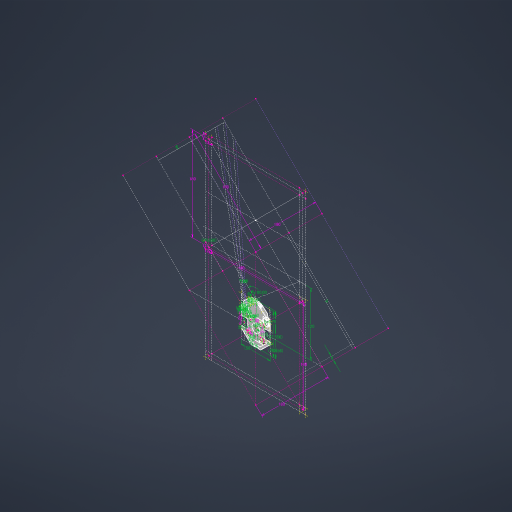
# Autodesk Inventor part: chassis
Saved by Autodesk Inventor 2023.5 (Build 275446000, 446)
## iProperties
Created: 2024-12-08
Part Number: chassis
Material: 一般
Document SubType Name: Modeling
Designer: IshiiLabHonda
Density: 1 g/cm^3
Appearance: 既定
Author: IshiiLabHonda
Autodesk Inventor part; units mm, degrees
(part 1 of 2)
ref_plane "YZ Plane" through (0, 0, 0) normal (1, 0, 0) x (0, 1, 0)
ref_plane "XZ Plane" through (0, 0, 0) normal (0, 1, 0) x (-1, 0, 0)
ref_plane "XY Plane" through (0, 0, 0) normal (0, 0, 1) x (1, 0, 0)
sketch "スケッチ1" plane through (0, 0, 0) normal (0, 0, 1) x (1, 0, 0)
  line L0 (0, 0) -> (0, 1) construction
  line L1 (0, 0) -> (1, 0) construction
  line L2 (-90, 90) -> (90, 90) construction
  line L3 (90, 90) -> (90, -90) construction
  line L4 (90, -90) -> (-90, -90) construction
  line L5 (-90, -90) -> (-90, 90) construction
  line L6 (-90, -90) -> (90, 90) construction
  line L7 (-90, 90) -> (90, -90) construction
  line L8 (-84, 96) -> (-84, 84) construction
  line L9 (-84, 84) -> (-96, 84) construction
  line L10 (-96, 84) -> (-96, 96) construction
  line L11 (-96, 96) -> (-84, 84) construction
  line L12 (-84, 96) -> (-96, 84) construction
  line L13 (-96, 96) -> (-84, 96) construction
  line L14 (-96, -96) -> (-96, -84) construction
  line L15 (-84, -96) -> (-96, -96) construction
  line L16 (-96, -96) -> (-84, -84) construction
  line L17 (-96, -84) -> (-84, -96) construction
  line L18 (-84, -84) -> (-84, -96) construction
  line L19 (-96, -84) -> (-84, -84) construction
  line L20 (96, -96) -> (84, -96) construction
  line L21 (96, -84) -> (96, -96) construction
  line L22 (96, -96) -> (84, -84) construction
  line L23 (84, -96) -> (96, -84) construction
  line L24 (84, -84) -> (96, -84) construction
  line L25 (84, -96) -> (84, -84) construction
  line L26 (96, 96) -> (96, 84) construction
  line L27 (84, 96) -> (96, 96) construction
  line L28 (96, 96) -> (84, 84) construction
  line L29 (96, 84) -> (84, 96) construction
  line L30 (84, 84) -> (84, 96) construction
  line L31 (96, 84) -> (84, 84) construction
  line L32 (-84, 84) -> (-84, -84) construction
  line L33 (-96, 84) -> (-96, -84) construction
  line L34 (-84, -84) -> (84, -84) construction
  line L35 (-84, -96) -> (84, -96) construction
  line L36 (96, 84) -> (96, -84) construction
  line L37 (84, 84) -> (84, -84) construction
  line L38 (-84, 96) -> (84, 96) construction
  line L39 (-84, 84) -> (84, 84) construction
  line L40 (-16, 15) -> (16, 15) construction
  line L41 (16, 15) -> (16, -15) construction
  line L42 (16, -15) -> (-16, -15) construction
  line L43 (-16, -15) -> (-16, 15) construction
  line L44 (-16, 15) -> (16, -15) construction
  line L45 (16, 15) -> (-16, -15) construction
  line L46 (-27.25, 11.5) -> (-16, 11.5) construction
  line L47 (-16, -11.5) -> (-27.25, -11.5) construction
  line L48 (-27.25, -11.5) -> (-27.25, 11.5) construction
  line L49 (-27.25, 11.5) -> (-16, -11.5) construction
  line L50 (-16, 11.5) -> (-27.25, -11.5) construction
  line L51 (27.25, 11.5) -> (16, 11.5) construction
  line L52 (16, -11.5) -> (27.25, -11.5) construction
  line L53 (27.25, -11.5) -> (27.25, 11.5) construction
  line L54 (27.25, 11.5) -> (16, -11.5) construction
  line L55 (16, 11.5) -> (27.25, -11.5) construction
  line L56 (-16, -10) -> (16, -10) construction
  line L57 (-16, -12.5) -> (16, -12.5) construction
  line L58 (-16, 10) -> (16, 10) construction
  line L59 (-16, 12.5) -> (16, 12.5) construction
  line L60 (-13.5, -15) -> (-13.5, 15) construction
  line L61 (13.5, -15) -> (13.5, 15) construction
  line L62 (-9.5, -10) -> (-9.5, -15) construction
  line L63 (-13.5, -10) -> (-9.5, -15) construction
  line L64 (-13.5, -15) -> (-9.5, -10) construction
  circle A0 centre (-11.5, -12.5) radius 0.8 construction
  line L65 (9.5, -10) -> (9.5, -15) construction
  line L66 (13.5, -10) -> (9.5, -15) construction
  line L67 (13.5, -15) -> (9.5, -10) construction
  circle A1 centre (11.5, -12.5) radius 0.8 construction
  line L68 (-9.5, 10) -> (-9.5, 15) construction
  line L69 (-13.5, 10) -> (-9.5, 15) construction
  line L70 (-13.5, 15) -> (-9.5, 10) construction
  circle A2 centre (-11.5, 12.5) radius 0.8 construction
  line L71 (9.5, 10) -> (9.5, 15) construction
  line L72 (13.5, 10) -> (9.5, 15) construction
  circle A3 centre (11.5, 12.5) radius 0.8 construction
  line L73 (13.5, 15) -> (9.5, 10) construction
  line L74 (-96, 276) -> (-84, 276) construction
  line L75 (-84, 276) -> (-84, 264) construction
  line L76 (-84, 264) -> (-96, 264) construction
  line L77 (-96, 264) -> (-96, 276) construction
  line L78 (-96, 276) -> (-84, 264) construction
  line L79 (-84, 276) -> (-96, 264) construction
  line L80 (-90, 90) -> (-90, 270) construction
  line L81 (-96, 264) -> (-96, 96) construction
  line L82 (-84, 264) -> (-84, 96) construction
  line L83 (96, 276) -> (84, 276) construction
  line L84 (84, 276) -> (84, 264) construction
  line L85 (84, 264) -> (96, 264) construction
  line L86 (96, 264) -> (96, 276) construction
  line L87 (96, 276) -> (84, 264) construction
  line L88 (84, 276) -> (96, 264) construction
  line L89 (90, 90) -> (90, 270) construction
  line L90 (96, 264) -> (96, 96) construction
  line L91 (84, 264) -> (84, 96) construction
  line L92 (-84, 276) -> (84, 276) construction
  line L93 (-84, 264) -> (84, 264) construction
  line L94 (-90, 270) -> (90, 270) construction
  line L95 (-90, 270) -> (90, 90) construction
  line L96 (-90, 90) -> (90, 270) construction
  circle A4 centre (0, 0) radius 15 construction
  line L97 (-96, 120) -> (96, 120) construction
  line L98 (0, 127.2792) -> (0, -127.2792) construction
  line L99 (-127.2792, 0) -> (127.2792, 0) construction
  line L100 (127.2792, 0) -> (0, -127.2792) construction
  line L101 (0, -127.2792) -> (-127.2792, 0) construction
  line L102 (-127.2792, 0) -> (0, 127.2792) construction
  line L103 (0, 127.2792) -> (127.2792, 0) construction
  line L104 (127.2792, 254.5584) -> (254.5584, 127.2792) construction
  line L105 (254.5584, 127.2792) -> (127.2792, 0) construction
  line L106 (127.2792, 0) -> (0, 127.2792) construction
  line L107 (0, 127.2792) -> (127.2792, 254.5584) construction
  line L108 (-127.2792, 254.5584) -> (0, 127.2792) construction
  line L109 (0, 127.2792) -> (-127.2792, 0) construction
  line L110 (-127.2792, 0) -> (-254.5584, 127.2792) construction
  line L111 (-254.5584, 127.2792) -> (-127.2792, 254.5584) construction
  line L112 (0, 381.8377) -> (127.2792, 254.5584) construction
  line L113 (127.2792, 254.5584) -> (0, 127.2792) construction
  line L114 (0, 127.2792) -> (-127.2792, 254.5584) construction
  line L115 (-127.2792, 254.5584) -> (0, 381.8377) construction
  line L116 (190.9188, 63.6396) -> (63.6396, 190.9188) construction
  line L117 (-190.9188, 190.9188) -> (-63.6396, 63.6396) construction
  line L118 (59.397, -59.397) -> (186.6762, 67.8823) construction
  line L119 (59.397, 186.6762) -> (186.6762, 59.397) construction
  line L120 (63.6396, 190.9188) -> (-63.6396, 318.1981) construction
  line L121 (-186.6762, 186.6762) -> (-59.397, 313.9554) construction
  point P0 (-90, -90)
  point P1 (90, -90)
  point P2 (-21.625, 0)
  point P3 (-84, 120)
  point P4 (84, 120)
  point P5 (0, 0)
  dimension "d0" = 1
  dimension "d1" = 1
  dimension "d2" = 180
  dimension "d3" = 180
  dimension "d4" = 12
  dimension "d5" = 12
  dimension "d8" = 360
  dimension "d10" = 32
  dimension "d12" = 11.25
  dimension "d13" = 23
  dimension "d14" = 5
  dimension "d15" = 2.5
  dimension "d16" = 4
  dimension "d17" = 1.6
  dimension "d22" = 12
  dimension "d23" = 12
  dimension "d24" = 180
  dimension "d25" = 25
  dimension "d26" = 30
  dimension "d27" = 30
  dimension "d29" = 120
  dimension "d331" = 180
  dimension "d334" = 180
  dimension "d337" = 180
  dimension "d340" = 6
  dimension "d341" = 6
  dimension "d342" = 6
  dimension "d561" = 27
  constraints: 244 end point, 29 point on line, 27 symmetric about line, 19 midpoint, 18 parallel, 10 perpendicular, 5 centre point, 4 coincident, 2 collinear, 1 horizontal, 1 vertical, 91 other
  measures "d0" distance of L0.start L0.end
  measures "d1" distance of L0.start L1.end
  measures "d2" distance of L2.start L2.end
  measures "d3" distance of L2.end L3.end
  measures "d4" distance of L9.end L10.end
  measures "d5" distance of L8.end L9.end
  measures "d10" distance of L40.start L40.end
  measures "d12" distance of L46.start L46.end
  measures "d13" distance of L47.end L46.start
  measures "d14" distance between parallel lines of L56 L42
  measures "d15" distance between parallel lines of L43 L60
  measures "d16" distance between parallel lines of L60 L62
  measures "d17" diameter of A0
  measures "d22" distance of L75.end L76.end
  measures "d23" distance of L76.end L74.start
  measures "d24" distance of L2.start L80.end
  measures "d25" distance between parallel lines of L57 L59
  measures "d26" distance between parallel lines of L42 L40
  measures "d27" diameter of A4
  measures "d29" distance between parallel lines of L1 L97
  measures "d331" distance of L100.start L100.end
  measures "d334" distance of L102.end L104.start
  measures "d337" distance of L102.end L108.start
  measures "d340" distance between parallel lines of L118 L105
  measures "d341" distance between parallel lines of L116 L119
  measures "d342" distance between parallel lines of L111 L121
  measures "d561" distance between parallel lines of L61 L60
sketch "スケッチ4" plane through (0, 0, 0) normal (0, 0, 1) x (1, 0, 0)
  line L0 (-84, 264) -> (-96, 264) construction
  line L1 (-90, 90) -> (-90, 270) construction
  line L2 (-96, 264) -> (-96, 96) construction
  line L3 (-96, 96) -> (-84, 96) construction
  line L4 (-84, 96) -> (-84, 84) construction
  line L5 (-84, 96) -> (-96, 84) construction
  line L6 (-96, 96) -> (-84, 84) construction
  line L7 (-84, 264) -> (-84, 96) construction
  line L8 (-84, 84) -> (-96, 84) construction
  line L9 (84, -84) -> (96, -84) construction
  line L10 (84, -96) -> (96, -84) construction
  line L11 (96, -96) -> (84, -84) construction
  line L12 (96, -84) -> (96, -96) construction
  line L13 (96, -96) -> (84, -96) construction
  line L14 (0, 0) -> (0, 1) construction
  line L15 (0, 0) -> (1, 0) construction
  line L16 (13.5, 15) -> (9.5, 10) construction
  line L17 (-96, 84) -> (-96, -84) construction
  line L18 (-84, 84) -> (-84, -84) construction
  line L19 (-90, -90) -> (-90, 90) construction
  line L20 (-90, 90) -> (90, 90) construction
  line L21 (-84, -84) -> (84, -84) construction
  line L22 (-84, -96) -> (84, -96) construction
  line L23 (-90, -90) -> (90, 90) construction
  line L24 (90, -90) -> (-90, -90) construction
  line L25 (-90, 90) -> (90, -90) construction
  line L26 (84, 84) -> (84, -84) construction
  line L27 (90, 90) -> (90, -90) construction
  line L28 (96, 84) -> (96, -84) construction
  line L29 (-96, 84) -> (-96, 96) construction
  line L30 (-84, -84) -> (-84, -96) construction
  line L31 (-96, -84) -> (-84, -84) construction
  line L32 (-84, -96) -> (-96, -96) construction
  line L33 (-96, -96) -> (-84, -84) construction
  line L34 (-96, -84) -> (-84, -96) construction
  line L35 (-96, -96) -> (-96, -84) construction
  line L36 (84, -96) -> (84, -84) construction
  line L37 (-16, -15) -> (-16, 15) construction
  line L38 (-27.25, 11.5) -> (-16, 11.5) construction
  line L39 (-16, -11.5) -> (-27.25, -11.5) construction
  line L40 (-16, 11.5) -> (-27.25, -11.5) construction
  line L41 (-27.25, 11.5) -> (-16, -11.5) construction
  line L42 (-27.25, -11.5) -> (-27.25, 11.5) construction
  line L43 (9.5, 10) -> (9.5, 15) construction
  circle A0 centre (11.5, 12.5) radius 0.8 construction
  line L44 (27.25, 11.5) -> (16, 11.5) construction
  line L45 (13.5, 10) -> (9.5, 15) construction
  circle A1 centre (11.5, -12.5) radius 0.8 construction
  line L46 (13.5, -15) -> (9.5, -10) construction
  line L47 (13.5, -10) -> (9.5, -15) construction
  line L48 (9.5, -10) -> (9.5, -15) construction
  circle A2 centre (-11.5, -12.5) radius 0.8 construction
  line L49 (-9.5, -10) -> (-9.5, -15) construction
  line L50 (-13.5, -15) -> (-9.5, -10) construction
  line L51 (-13.5, -10) -> (-9.5, -15) construction
  line L52 (96, 84) -> (84, 84) construction
  line L53 (96, 96) -> (96, 84) construction
  line L54 (84, 96) -> (96, 96) construction
  line L55 (96, 96) -> (84, 84) construction
  line L56 (84, 84) -> (84, 96) construction
  line L57 (96, 84) -> (84, 96) construction
  line L58 (-96, 264) -> (-96, 276) construction
  line L59 (-84, 276) -> (-84, 264) construction
  line L60 (-96, 276) -> (-84, 276) construction
  line L61 (-96, 276) -> (-84, 264) construction
  line L62 (-84, 276) -> (-96, 264) construction
  line L63 (-84, 84) -> (84, 84) construction
  line L64 (-84, 96) -> (84, 96) construction
  line L65 (84, 264) -> (84, 96) construction
  line L66 (90, 90) -> (90, 270) construction
  line L67 (-90, 90) -> (90, 270) construction
  line L68 (-90, 270) -> (90, 90) construction
  line L69 (96, 264) -> (96, 96) construction
  line L70 (-96, 120) -> (96, 120) construction
  line L71 (-84, 264) -> (84, 264) construction
  line L72 (-84, 276) -> (84, 276) construction
  line L73 (-90, 270) -> (90, 270) construction
  line L74 (84, 276) -> (84, 264) construction
  line L75 (84, 264) -> (96, 264) construction
  line L76 (96, 264) -> (96, 276) construction
  line L77 (96, 276) -> (84, 264) construction
  line L78 (96, 276) -> (84, 276) construction
  line L79 (84, 276) -> (96, 264) construction
  line L80 (-16, 15) -> (16, 15) construction
  line L81 (16, 15) -> (16, -15) construction
  line L82 (16, -15) -> (-16, -15) construction
  circle A3 centre (-11.5, 12.5) radius 0.8 construction
  line L83 (-13.5, 10) -> (-9.5, 15) construction
  line L84 (-9.5, 10) -> (-9.5, 15) construction
  line L85 (-13.5, 15) -> (-9.5, 10) construction
  circle A4 centre (0, 0) radius 15 construction
  line L86 (-16, 10) -> (16, 10) construction
  line L87 (-16, 12.5) -> (16, 12.5) construction
  line L88 (-16, 15) -> (16, -15) construction
  line L89 (16, 15) -> (-16, -15) construction
  line L90 (-16, -10) -> (16, -10) construction
  line L91 (-16, -12.5) -> (16, -12.5) construction
  line L92 (13.5, -15) -> (13.5, 15) construction
  line L93 (16, 11.5) -> (27.25, -11.5) construction
  line L94 (16, -11.5) -> (27.25, -11.5) construction
  line L95 (27.25, -11.5) -> (27.25, 11.5) construction
  line L96 (27.25, 11.5) -> (16, -11.5) construction
  line L97 (-13.5, -15) -> (-13.5, 15) construction
  line L98 (-84, 120) -> (27.25, 26.6502) construction
  line L99 (84, 120) -> (-27.25, 26.6502) construction
  line L100 (-27.25, 45) -> (27.25, 45) construction
  line L101 (0.8414, 45) -> (-27.25, 21.4285) construction
  line L102 (-0.8414, 45) -> (27.25, 21.4285) construction
  line L103 (-11.6044, 45) -> (-27.25, 31.8718) construction
  line L104 (-8.9719, 46.5563) -> (-4.4723, 41.194) construction
  line L105 (-4.4723, 41.194) -> (-9.4516, 37.0158) construction
  line L106 (-9.4516, 37.0158) -> (-13.9511, 42.3782) construction
  line L107 (-13.9511, 42.3782) -> (-8.9719, 46.5563) construction
  line L108 (-8.9719, 46.5563) -> (-9.4516, 37.0158) construction
  line L109 (-4.4723, 41.194) -> (-13.9511, 42.3782) construction
  line L110 (-8.3291, 45.7902) -> (-13.3084, 41.6121) construction
  line L111 (-5.1151, 41.96) -> (-10.0944, 37.7819) construction
  line L112 (-9.2117, 41.7861) -> (-8.5989, 42.3003) construction
  line L113 (-9.2117, 41.7861) -> (-8.6975, 41.1732) construction
  line L114 (-9.0269, 43.8993) -> (-7.0985, 41.6012) construction
  line L115 (-7.0985, 41.6012) -> (-9.3966, 39.6728) construction
  line L116 (-9.3966, 39.6728) -> (-11.325, 41.9709) construction
  line L117 (-11.325, 41.9709) -> (-9.0269, 43.8993) construction
  line L118 (-9.0269, 43.8993) -> (-9.3966, 39.6728) construction
  line L119 (-7.0985, 41.6012) -> (-11.325, 41.9709) construction
  circle A5 centre (-9.2117, 41.7861) radius 0.8 construction
  line L120 (-27.25, 11.5) -> (-27.25, 45) construction
  line L121 (27.25, 11.5) -> (27.25, 45) construction
  line L122 (-11.0762, 35) -> (11.0762, 35) construction
  line L123 (-28, 45) -> (-28, -31) construction
  line L124 (28, 45) -> (28, -31) construction
  line L125 (-27.25, 45) -> (-28, 45) construction
  line L126 (27.25, 45) -> (28, 45) construction
  line L127 (-28, 8.5) -> (28, 8.5) construction
  line L128 (-28, -8.5) -> (28, -8.5) construction
  circle A6 centre (0, 0) radius 7.5 construction
  line L129 (-28, -31) -> (28, -31) construction
  line L130 (-27.25, 31.8718) -> (-28, 31.2425) construction
  line L131 (-27.25, 21.4285) -> (-28, 20.7992) construction
  line L132 (-22.25, 21.5) -> (-22.3613, 22.2922) construction
  line L133 (-22.25, 21.5) -> (-21.4578, 21.6113) construction
  line L134 (-25.0736, 23.6277) -> (-20.1223, 24.3236) construction
  line L135 (-20.1223, 24.3236) -> (-19.4264, 19.3723) construction
  line L136 (-19.4264, 19.3723) -> (-24.3777, 18.6764) construction
  line L137 (-24.3777, 18.6764) -> (-25.0736, 23.6277) construction
  line L138 (-25.0736, 23.6277) -> (-19.4264, 19.3723) construction
  line L139 (-20.1223, 24.3236) -> (-24.3777, 18.6764) construction
  circle A7 centre (-22.25, 21.5) radius 0.8 construction
  line L140 (-22.25, 45) -> (-22.25, -31) construction
  line L141 (-96, 180) -> (96, 180) construction
  line L142 (-22.3613, 22.2922) -> (-62.8646, 310.4878) construction
  line L143 (-186.6762, 186.6762) -> (-59.397, 313.9554) construction
  line L144 (59.397, 186.6762) -> (186.6762, 59.397) construction
  line L145 (-22.25, 21.5) -> (-77.9717, 295.3807) construction
  line L146 (-22.25, 21.5) -> (-44.0597, 298.6181) construction
  line L147 (63.6396, 190.9188) -> (-63.6396, 318.1981) construction
  line L148 (8.9719, 46.5563) -> (4.4723, 41.194) construction
  line L149 (4.4723, 41.194) -> (9.4516, 37.0158) construction
  line L150 (9.4516, 37.0158) -> (13.9511, 42.3782) construction
  line L151 (13.9511, 42.3782) -> (8.9719, 46.5563) construction
  line L152 (8.9719, 46.5563) -> (9.4516, 37.0158) construction
  line L153 (4.4723, 41.194) -> (13.9511, 42.3782) construction
  line L154 (8.3291, 45.7902) -> (13.3084, 41.6121) construction
  line L155 (5.1151, 41.96) -> (10.0944, 37.7819) construction
  line L156 (9.2117, 41.7861) -> (8.5989, 42.3003) construction
  line L157 (9.2117, 41.7861) -> (8.6975, 41.1732) construction
  line L158 (9.0269, 43.8993) -> (7.0985, 41.6012) construction
  line L159 (7.0985, 41.6012) -> (9.3966, 39.6728) construction
  line L160 (9.3966, 39.6728) -> (11.325, 41.9709) construction
  line L161 (11.325, 41.9709) -> (9.0269, 43.8993) construction
  line L162 (9.0269, 43.8993) -> (9.3966, 39.6728) construction
  line L163 (7.0985, 41.6012) -> (11.325, 41.9709) construction
  circle A8 centre (9.2117, 41.7861) radius 0.8 construction
  line L164 (-20.1223, 24.3236) -> (-15.1709, 25.0195) construction
  line L165 (-15.1709, 25.0195) -> (-14.4751, 20.0681) construction
  line L166 (-14.4751, 20.0681) -> (-19.4264, 19.3723) construction
  line L167 (-20.1223, 24.3236) -> (-25.0736, 23.6277) construction
  line L168 (-25.0736, 23.6277) -> (-24.3777, 18.6764) construction
  line L169 (-24.3777, 18.6764) -> (-19.4264, 19.3723) construction
  line L170 (24.3777, 18.6764) -> (25.0736, 23.6277) construction
  line L171 (20.1223, 24.3236) -> (15.1709, 25.0195) construction
  line L172 (15.1709, 25.0195) -> (14.4751, 20.0681) construction
  line L173 (14.4751, 20.0681) -> (19.4264, 19.3723) construction
  line L174 (20.1223, 24.3236) -> (25.0736, 23.6277) construction
  line L175 (25.0736, 23.6277) -> (24.3777, 18.6764) construction
  line L176 (24.3777, 18.6764) -> (19.4264, 19.3723) construction
  line L177 (20.1223, 24.3236) -> (24.3777, 18.6764) construction
  line L178 (19.4264, 19.3723) -> (25.0736, 23.6277) construction
  line L179 (-17.2987, 22.1959) -> (-58.4376, 314.9148) construction
  line L180 (-17.2987, 22.1959) -> (-73.7397, 299.6126) construction
  line L181 (-17.2987, 22.1959) -> (-38.6259, 293.1844) construction
  line L182 (-20.1223, 24.3236) -> (-14.4751, 20.0681) construction
  line L183 (-19.4264, 19.3723) -> (-15.1709, 25.0195) construction
  line L184 (-13.9511, 42.3782) -> (-16.2493, 40.4498) construction
  line L185 (-16.2493, 40.4498) -> (-11.7498, 35.0875) construction
  line L186 (-11.7498, 35.0875) -> (-9.4516, 37.0158) construction
  point P0 (90, -90)
  point P1 (-90, -90)
  point P2 (-21.625, 0)
  point P3 (0, 49.5156)
  point P4 (-5.3815, 45)
  point P5 (-6.7221, 43.8751)
  point P6 (0, 180)
  point P7 (6.7221, 43.8751)
  dimension "d264" = 100
  dimension "d275" = 7
  dimension "d276" = 6.5
  dimension "d277" = 5
  dimension "d278" = 3
  dimension "d279" = 3
  dimension "d280" = 1.6
  dimension "d281" = 8
  dimension "d284" = 10
  dimension "d288" = 17
  dimension "d289" = 15
  dimension "d290" = 0.75
  dimension "d291" = 0.75
  dimension "d292" = 76
  dimension "d296" = 5
  dimension "d297" = 5
  dimension "d298" = 1.6
  dimension "d299" = 8
  dimension "d345" = 7
  dimension "d346" = 10
  dimension "d356" = 16
  dimension "d367" = 5
  dimension "d369" = 30
  dimension "d370" = 5
  dimension "d371" = 56
  dimension "d382" = 5
  dimension "d385" = 7
  dimension "d513" = 3
  constraints: 172 end point, 38 point on line, 25 symmetric about line, 19 parallel, 15 perpendicular, 13 midpoint, 6 point on circle, 5 collinear, 4 centre point, 4 coincident, 2 equal length, 8 other
  measures "d264" angle of L99 L98
  measures "d275" distance of L104.start L104.end
  measures "d276" distance of L106.end L104.start
  measures "d277" distance between parallel lines of L110 L111
  measures "d278" distance of L115.end L116.end
  measures "d279" distance of L114.end L115.end
  measures "d280" diameter of A5
  measures "d281" distance between parallel lines of L101 L103
  measures "d284" distance between parallel lines of L100 L122
  measures "d288" distance between parallel lines of L128 L127
  measures "d289" diameter of A6
  measures "d290" distance between parallel lines of L123 L120
  measures "d291" distance between parallel lines of L121 L124
  measures "d292" distance between parallel lines of L129 L100
  measures "d296" distance of L135.end L136.end
  measures "d297" distance of L134.end L135.end
  measures "d298" diameter of A7
  measures "d299" angle of L140 L132
  measures "d345" angle of L145 L146
  measures "d346" distance from line of L38 L132.start
  measures "d356" distance between parallel lines of L129 L82
  measures "d367" distance between parallel lines of L120 L140
  measures "d369" distance between parallel lines of L80 L100
  measures "d370" distance of L112.start point (-5.382, 45)
  measures "d371" distance of L123.end L124.end
  measures "d382" distance of L134.end L164.end
  measures "d385" angle of L180 L181
  measures "d513" distance between parallel lines of L185 L106
sketch "スケッチ5" plane through (0, 0, 0) normal (0, 0, 1) x (1, 0, 0)
  line L0 (0, 0) -> (0, 1) construction
  line L1 (27.25, 11.5) -> (16, 11.5) construction
  line L2 (16, 11.5) -> (27.25, -11.5) construction
  line L3 (27.25, 11.5) -> (16, -11.5) construction
  line L4 (27.25, -11.5) -> (27.25, 11.5) construction
  line L5 (16, -11.5) -> (27.25, -11.5) construction
  line L6 (-90, 90) -> (90, 90) construction
  line L7 (-90, -90) -> (90, 90) construction
  line L8 (-90, 90) -> (90, -90) construction
  line L9 (-84, 84) -> (-84, -84) construction
  line L10 (-96, 84) -> (-96, -84) construction
  line L11 (-90, -90) -> (-90, 90) construction
  line L12 (-84, 84) -> (-96, 84) construction
  line L13 (-96, 84) -> (-96, 96) construction
  line L14 (84, 84) -> (84, -84) construction
  line L15 (90, 90) -> (90, -90) construction
  line L16 (96, 84) -> (84, 84) construction
  line L17 (96, 84) -> (96, -84) construction
  line L18 (90, -90) -> (-90, -90) construction
  line L19 (-84, -84) -> (84, -84) construction
  line L20 (-84, -96) -> (84, -96) construction
  line L21 (-84, -84) -> (-84, -96) construction
  line L22 (-96, -96) -> (-96, -84) construction
  line L23 (-84, -96) -> (-96, -96) construction
  line L24 (-96, -96) -> (-84, -84) construction
  line L25 (-96, -84) -> (-84, -96) construction
  line L26 (-96, -84) -> (-84, -84) construction
  line L27 (0, 0) -> (1, 0) construction
  line L28 (-84, 264) -> (-96, 264) construction
  line L29 (-96, 276) -> (-84, 276) construction
  line L30 (-96, 264) -> (-96, 276) construction
  line L31 (-84, 276) -> (-96, 264) construction
  line L32 (-96, 276) -> (-84, 264) construction
  line L33 (-84, 276) -> (-84, 264) construction
  line L34 (84, -96) -> (84, -84) construction
  line L35 (96, -96) -> (84, -96) construction
  line L36 (96, -84) -> (96, -96) construction
  line L37 (96, -96) -> (84, -84) construction
  line L38 (84, -96) -> (96, -84) construction
  line L39 (84, -84) -> (96, -84) construction
  line L40 (-16, 15) -> (16, 15) construction
  line L41 (16, 15) -> (16, -15) construction
  line L42 (13.5, 15) -> (9.5, 10) construction
  line L43 (9.5, 10) -> (9.5, 15) construction
  line L44 (13.5, 10) -> (9.5, 15) construction
  line L45 (13.5, -15) -> (13.5, 15) construction
  line L46 (-16, 10) -> (16, 10) construction
  line L47 (-16, 12.5) -> (16, 12.5) construction
  circle A0 centre (0, 0) radius 15 construction
  line L48 (-16, -10) -> (16, -10) construction
  line L49 (-16, -12.5) -> (16, -12.5) construction
  line L50 (16, -15) -> (-16, -15) construction
  line L51 (-16, 15) -> (16, -15) construction
  line L52 (16, 15) -> (-16, -15) construction
  line L53 (-13.5, -15) -> (-13.5, 15) construction
  line L54 (-16, -15) -> (-16, 15) construction
  line L55 (-27.25, 11.5) -> (-16, 11.5) construction
  line L56 (-16, -11.5) -> (-27.25, -11.5) construction
  line L57 (-27.25, -11.5) -> (-27.25, 11.5) construction
  line L58 (-27.25, 11.5) -> (-16, -11.5) construction
  line L59 (-16, 11.5) -> (-27.25, -11.5) construction
  line L60 (-9.5, 10) -> (-9.5, 15) construction
  circle A1 centre (-11.5, 12.5) radius 0.8 construction
  line L61 (-13.5, 10) -> (-9.5, 15) construction
  line L62 (-13.5, 15) -> (-9.5, 10) construction
  circle A2 centre (11.5, 12.5) radius 0.8 construction
  line L63 (-84, 96) -> (-96, 84) construction
  line L64 (-96, 96) -> (-84, 96) construction
  line L65 (-84, 96) -> (-84, 84) construction
  line L66 (-96, 96) -> (-84, 84) construction
  line L67 (-96, 264) -> (-96, 96) construction
  line L68 (-84, 264) -> (-84, 96) construction
  line L69 (-84, 96) -> (84, 96) construction
  line L70 (-84, 84) -> (84, 84) construction
  line L71 (84, 84) -> (84, 96) construction
  line L72 (96, 96) -> (96, 84) construction
  line L73 (96, 96) -> (84, 84) construction
  line L74 (96, 84) -> (84, 96) construction
  line L75 (-96, 120) -> (96, 120) construction
  line L76 (84, 96) -> (96, 96) construction
  line L77 (-84, 264) -> (84, 264) construction
  line L78 (84, 264) -> (84, 96) construction
  line L79 (-84, 276) -> (84, 276) construction
  line L80 (96, 264) -> (96, 96) construction
  line L81 (-90, 270) -> (90, 270) construction
  line L82 (-90, 270) -> (90, 90) construction
  line L83 (-90, 90) -> (90, 270) construction
  line L84 (90, 90) -> (90, 270) construction
  line L85 (-90, 90) -> (-90, 270) construction
  line L86 (84, 264) -> (96, 264) construction
  line L87 (96, 276) -> (84, 276) construction
  line L88 (96, 276) -> (84, 264) construction
  line L89 (84, 276) -> (96, 264) construction
  line L90 (96, 264) -> (96, 276) construction
  line L91 (84, 276) -> (84, 264) construction
  circle A3 centre (-11.5, -12.5) radius 0.8 construction
  line L92 (-9.5, -10) -> (-9.5, -15) construction
  line L93 (-13.5, -15) -> (-9.5, -10) construction
  line L94 (9.5, -10) -> (9.5, -15) construction
  circle A4 centre (11.5, -12.5) radius 0.8 construction
  line L95 (13.5, -15) -> (9.5, -10) construction
  line L96 (13.5, -10) -> (9.5, -15) construction
  line L97 (-13.5, -10) -> (-9.5, -15) construction
  line L98 (-11.325, 41.9709) -> (-9.0269, 43.8993) construction
  line L99 (-7.0985, 41.6012) -> (-11.325, 41.9709) construction
  circle A5 centre (-9.2117, 41.7861) radius 0.8 construction
  line L100 (-7.0985, 41.6012) -> (-9.3966, 39.6728) construction
  line L101 (-9.0269, 43.8993) -> (-9.3966, 39.6728) construction
  line L102 (-9.3966, 39.6728) -> (-11.325, 41.9709) construction
  line L103 (-27.25, 31.8718) -> (-28, 31.2425) construction
  line L104 (-11.6044, 45) -> (-27.25, 31.8718) construction
  line L105 (-27.25, 45) -> (-28, 45) construction
  line L106 (-9.0269, 43.8993) -> (-7.0985, 41.6012) construction
  line L107 (-27.25, 45) -> (27.25, 45) construction
  line L108 (-4.4723, 41.194) -> (-9.4516, 37.0158) construction
  line L109 (-9.4516, 37.0158) -> (-13.9511, 42.3782) construction
  line L110 (-8.9719, 46.5563) -> (-4.4723, 41.194) construction
  line L111 (0.8414, 45) -> (-27.25, 21.4285) construction
  line L112 (-0.8414, 45) -> (27.25, 21.4285) construction
  line L113 (-16, 15) -> (16, 15) construction
  line L114 (9.5, 10) -> (9.5, 15) construction
  line L115 (-16, 10) -> (16, 10) construction
  circle A6 centre (-11.5, 12.5) radius 0.8 construction
  line L116 (-9.5, 10) -> (-9.5, 15) construction
  line L117 (-13.5, 10) -> (-9.5, 15) construction
  line L118 (-13.5, 15) -> (-9.5, 10) construction
  line L119 (-16, 12.5) -> (16, 12.5) construction
  line L120 (27.25, 45) -> (28, 45) construction
  line L121 (27.25, 11.5) -> (27.25, 45) construction
  line L122 (-11.0762, 35) -> (11.0762, 35) construction
  line L123 (-27.25, 21.4285) -> (-28, 20.7992) construction
  line L124 (-27.25, 11.5) -> (-27.25, 45) construction
  line L125 (-5.1151, 41.96) -> (-10.0944, 37.7819) construction
  line L126 (-9.2117, 41.7861) -> (-8.6975, 41.1732) construction
  line L127 (-9.2117, 41.7861) -> (-8.5989, 42.3003) construction
  line L128 (-4.4723, 41.194) -> (-13.9511, 42.3782) construction
  line L129 (-8.3291, 45.7902) -> (-13.3084, 41.6121) construction
  line L130 (-13.9511, 42.3782) -> (-8.9719, 46.5563) construction
  line L131 (-8.9719, 46.5563) -> (-9.4516, 37.0158) construction
  line L132 (-27.25, 11.5) -> (-16, 11.5) construction
  line L133 (-27.25, 11.5) -> (-16, -11.5) construction
  line L134 (27.25, 11.5) -> (16, 11.5) construction
  line L135 (27.25, -11.5) -> (27.25, 11.5) construction
  line L136 (16, 11.5) -> (27.25, -11.5) construction
  line L137 (27.25, 11.5) -> (16, -11.5) construction
  line L138 (0, 0) -> (0, 1) construction
  line L139 (0, 0) -> (1, 0) construction
  circle A7 centre (0, 0) radius 7.5 construction
  circle A8 centre (0, 0) radius 15 construction
  line L140 (-13.5, -15) -> (-13.5, 15) construction
  circle A9 centre (11.5, 12.5) radius 0.8 construction
  line L141 (-9.5, -10) -> (-9.5, -15) construction
  line L142 (9.5, -10) -> (9.5, -15) construction
  line L143 (13.5, 10) -> (9.5, 15) construction
  line L144 (-13.5, -15) -> (-9.5, -10) construction
  line L145 (13.5, -10) -> (9.5, -15) construction
  line L146 (13.5, 15) -> (9.5, 10) construction
  line L147 (-16, -12.5) -> (16, -12.5) construction
  line L148 (16, -15) -> (-16, -15) construction
  line L149 (-16, 11.5) -> (-27.25, -11.5) construction
  line L150 (16, -11.5) -> (27.25, -11.5) construction
  line L151 (-16, -11.5) -> (-27.25, -11.5) construction
  line L152 (-27.25, -11.5) -> (-27.25, 11.5) construction
  line L153 (13.5, -15) -> (13.5, 15) construction
  line L154 (16, 15) -> (16, -15) construction
  line L155 (-16, -15) -> (-16, 15) construction
  line L156 (-16, 15) -> (16, -15) construction
  line L157 (16, 15) -> (-16, -15) construction
  line L158 (-28, -8.5) -> (28, -8.5) construction
  line L159 (-28, 8.5) -> (28, 8.5) construction
  line L160 (-28, -31) -> (28, -31) construction
  line L161 (-28, 45) -> (-28, -31) construction
  line L162 (28, 45) -> (28, -31) construction
  line L163 (84, -84) -> (96, -84) construction
  line L164 (84, -96) -> (96, -84) construction
  line L165 (96, -96) -> (84, -84) construction
  line L166 (96, -84) -> (96, -96) construction
  line L167 (96, -96) -> (84, -96) construction
  line L168 (-96, 84) -> (-96, -84) construction
  line L169 (-84, 84) -> (-84, -84) construction
  line L170 (-90, -90) -> (-90, 90) construction
  line L171 (-84, -84) -> (84, -84) construction
  line L172 (-84, -96) -> (84, -96) construction
  line L173 (-90, -90) -> (90, 90) construction
  line L174 (90, -90) -> (-90, -90) construction
  line L175 (-90, 90) -> (90, -90) construction
  line L176 (84, 84) -> (84, -84) construction
  line L177 (90, 90) -> (90, -90) construction
  line L178 (96, 84) -> (96, -84) construction
  line L179 (84, -96) -> (84, -84) construction
  line L180 (-16, -10) -> (16, -10) construction
  circle A10 centre (11.5, -12.5) radius 0.8 construction
  line L181 (13.5, -15) -> (9.5, -10) construction
  line L182 (-13.5, -10) -> (-9.5, -15) construction
  line L183 (-84, -84) -> (-84, -96) construction
  line L184 (-96, -84) -> (-84, -84) construction
  line L185 (-84, -96) -> (-96, -96) construction
  line L186 (-96, -96) -> (-84, -84) construction
  line L187 (-96, -84) -> (-84, -96) construction
  line L188 (-96, -96) -> (-96, -84) construction
  circle A11 centre (-11.5, -12.5) radius 0.8 construction
  line L189 (-96, 96) -> (-84, 96) construction
  line L190 (-84, 96) -> (-84, 84) construction
  line L191 (-84, 96) -> (-96, 84) construction
  line L192 (-96, 96) -> (-84, 84) construction
  line L193 (84, 96) -> (96, 96) construction
  line L194 (96, 84) -> (84, 84) construction
  line L195 (96, 96) -> (96, 84) construction
  line L196 (96, 96) -> (84, 84) construction
  line L197 (96, 84) -> (84, 96) construction
  line L198 (-96, 120) -> (96, 120) construction
  line L199 (-84, 96) -> (84, 96) construction
  line L200 (-90, 90) -> (90, 90) construction
  line L201 (-84, 84) -> (-96, 84) construction
  line L202 (-96, 84) -> (-96, 96) construction
  line L203 (-84, 84) -> (84, 84) construction
  line L204 (84, 120) -> (-27.25, 26.6502) construction
  line L205 (-84, 120) -> (27.25, 26.6502) construction
  line L206 (84, 84) -> (84, 96) construction
  line L207 (-84, 264) -> (-96, 264) construction
  line L208 (-90, 90) -> (-90, 270) construction
  line L209 (-96, 264) -> (-96, 96) construction
  line L210 (-84, 264) -> (-84, 96) construction
  line L211 (96, 264) -> (96, 96) construction
  line L212 (84, 264) -> (84, 96) construction
  line L213 (90, 90) -> (90, 270) construction
  line L214 (-90, 90) -> (90, 270) construction
  line L215 (-90, 270) -> (90, 90) construction
  line L216 (-84, 264) -> (84, 264) construction
  line L217 (-90, 270) -> (90, 270) construction
  line L218 (-96, 264) -> (-96, 276) construction
  line L219 (-96, 276) -> (-84, 276) construction
  line L220 (-96, 276) -> (-84, 264) construction
  line L221 (-84, 276) -> (-96, 264) construction
  line L222 (-84, 276) -> (-84, 264) construction
  line L223 (-84, 276) -> (84, 276) construction
  line L224 (84, 264) -> (96, 264) construction
  line L225 (96, 264) -> (96, 276) construction
  line L226 (96, 276) -> (84, 264) construction
  line L227 (96, 276) -> (84, 276) construction
  line L228 (84, 276) -> (96, 264) construction
  line L229 (84, 276) -> (84, 264) construction
  line L230 (-28, 8.5) -> (-16, 8.5)
  line L231 (-28, -8.5) -> (-16, -8.5)
  line L232 (-16, 8.5) -> (-16, -8.5)
  circle A12 centre (0, 0) radius 7.5
  line L233 (28, 8.5) -> (16, 8.5)
  line L234 (28, -8.5) -> (16, -8.5)
  line L235 (16, 8.5) -> (16, -8.5)
  line L236 (28, 8.5) -> (28, 8.5)
  line L237 (-28, -8.5) -> (-9.1203, -31) construction
  line L238 (-9.1203, -31) -> (9.1203, -31)
  line L239 (28, -8.5) -> (9.1203, -31) construction
  circle A13 centre (-11.5, 12.5) radius 1.05
  circle A14 centre (11.5, 12.5) radius 1.05
  circle A15 centre (-11.5, -12.5) radius 1.05
  circle A16 centre (11.5, -12.5) radius 1.05
  line L240 (-22.25, 21.5) -> (-22.3613, 22.2922) construction
  line L241 (-22.25, 21.5) -> (-21.4578, 21.6113) construction
  circle A17 centre (-22.25, 21.5) radius 0.8 construction
  line L242 (-20.1223, 24.3236) -> (-19.4264, 19.3723) construction
  line L243 (-24.3777, 18.6764) -> (-25.0736, 23.6277) construction
  line L244 (-20.1223, 24.3236) -> (-24.3777, 18.6764) construction
  line L245 (-25.0736, 23.6277) -> (-20.1223, 24.3236) construction
  line L246 (-19.4264, 19.3723) -> (-24.3777, 18.6764) construction
  line L247 (-25.0736, 23.6277) -> (-19.4264, 19.3723) construction
  line L248 (-25.0736, 23.6277) -> (-24.3777, 18.6764)
  line L249 (-20.1223, 24.3236) -> (-15.1709, 25.0195) construction
  line L250 (-15.1709, 25.0195) -> (-14.4751, 20.0681) construction
  line L251 (-14.4751, 20.0681) -> (-19.4264, 19.3723) construction
  line L252 (24.3777, 18.6764) -> (19.4264, 19.3723) construction
  line L253 (14.4751, 20.0681) -> (19.4264, 19.3723) construction
  line L254 (15.1709, 25.0195) -> (14.4751, 20.0681) construction
  line L255 (20.1223, 24.3236) -> (15.1709, 25.0195) construction
  line L256 (20.1223, 24.3236) -> (25.0736, 23.6277) construction
  line L257 (25.0736, 23.6277) -> (24.3777, 18.6764) construction
  line L258 (-25.0736, 23.6277) -> (-15.1709, 25.0195)
  line L259 (-14.4751, 20.0681) -> (-15.1709, 25.0195)
  line L260 (-14.4751, 20.0681) -> (-24.3777, 18.6764)
  line L261 (15.1709, 25.0195) -> (25.0736, 23.6277)
  line L262 (24.3777, 18.6764) -> (25.0736, 23.6277)
  line L263 (24.3777, 18.6764) -> (14.4751, 20.0681)
  line L264 (15.1709, 25.0195) -> (14.4751, 20.0681)
  line L265 (-8.558, 47.5563) -> (8.558, 47.5563)
  line L266 (-8.558, 47.5563) -> (-8.558, 47.5563)
  line L267 (-2.558, 47.5563) -> (0.1895, 46.5563)
  line L268 (0.1895, 46.5563) -> (-0.1895, 46.5563)
  line L269 (-0.1895, 46.5563) -> (2.558, 47.5563)
  line L270 (-3.6267, 42.5563) -> (3.6267, 42.5563)
  line L271 (-18.2592, 30.2781) -> (-3.6267, 42.5563)
  line L272 (-28, 8.5) -> (-22.1166, 36.1792)
  line L273 (-22.1166, 36.1792) -> (-8.558, 47.5563)
  line L274 (28, 8.5) -> (22.1166, 36.1792)
  line L275 (-18.2592, 30.2781) -> (-20.6565, 19)
  line L276 (18.2592, 30.2781) -> (20.6565, 19)
  line L277 (-20.6565, 19) -> (20.6565, 19)
  line L278 (-14.6308, -20) -> (14.6308, -20)
  line L279 (14.6308, -20) -> (8.5077, -26)
  line L280 (8.5077, -26) -> (-8.5077, -26)
  line L281 (-8.5077, -26) -> (-14.6308, -20)
  line L282 (-28, -8.5) -> (-28, -12.5)
  line L283 (-28, -12.5) -> (-9.1203, -31)
  line L284 (28, -8.5) -> (28, -12.5)
  line L285 (28, -12.5) -> (9.1203, -31)
  line L286 (-28, 8.5) -> (-28, 26.5)
  line L287 (-28, 26.5) -> (-23.3435, 30.4073)
  line L288 (28, 8.5) -> (28, 26.5)
  line L289 (28, 26.5) -> (23.3435, 30.4073)
  line L290 (-5.1203, -31) -> (-3.6203, -29.5)
  line L291 (-3.6203, -29.5) -> (3.6203, -29.5)
  line L292 (3.6203, -29.5) -> (5.1203, -31)
  line L293 (18.2592, 30.2781) -> (3.6267, 42.5563)
  line L294 (22.1166, 36.1792) -> (8.558, 47.5563)
  line L295 (-20.6565, 19) -> (-21.8255, 13.5)
  line L296 (-21.8255, 13.5) -> (-17.8255, 13.5)
  line L297 (-17.8255, 13.5) -> (-12.3255, 19)
  line L298 (20.6565, 19) -> (21.8255, 13.5)
  line L299 (21.8255, 13.5) -> (17.8255, 13.5)
  line L300 (17.8255, 13.5) -> (12.3255, 19)
  line L301 (-14.6308, -20) -> (-21.2643, -13.5)
  line L302 (-21.2643, -13.5) -> (-18.2643, -13.5)
  line L303 (-18.2643, -13.5) -> (-8.6308, -20)
  line L304 (14.6308, -20) -> (21.2643, -13.5)
  line L305 (21.2643, -13.5) -> (18.2643, -13.5)
  line L306 (18.2643, -13.5) -> (8.6308, -20)
  circle A18 centre (-7.1308, -17) radius 0.625 construction
  circle A19 centre (-7.1308, -17) radius 0.8
  circle A20 centre (-7.1308, -17) radius 1.5
  line L307 (-8.6308, -20) -> (-8.6308, -15) construction
  circle A21 centre (7.1308, -17) radius 0.625 construction
  circle A22 centre (7.1308, -17) radius 0.8
  circle A23 centre (7.1308, -17) radius 1.5
  circle A24 centre (-9, 15.5) radius 0.625 construction
  circle A25 centre (-9, 15.5) radius 0.8
  circle A26 centre (-9, 15.5) radius 1.5
  circle A27 centre (9, 15.5) radius 0.625 construction
  circle A28 centre (9, 15.5) radius 0.8
  circle A29 centre (9, 15.5) radius 1.5
  circle A30 centre (-21.1204, 28.8416) radius 0.8
  circle A31 centre (-21.1204, 28.8416) radius 1.5 construction
  circle A32 centre (21.1204, 28.8416) radius 0.475 construction
  circle A33 centre (21.1204, 28.8416) radius 0.8
  circle A34 centre (21.1204, 28.8416) radius 1.5 construction
  line L308 (-26.8721, 25.6471) -> (-13.9987, 27.4563)
  line L309 (-13.9987, 27.4563) -> (-12.6765, 18.0488)
  line L310 (-12.6765, 18.0488) -> (-25.55, 16.2395)
  line L311 (-25.55, 16.2395) -> (-26.8721, 25.6471)
  line L312 (-22.1166, 36.1792) -> (-18.2592, 30.2781) construction
  line L313 (-18.8107, 27.6837) -> (-23, 24.1685)
  line L314 (-23, 24.1685) -> (-23, 13.5)
  line L315 (-21.8255, 13.5) -> (-23, 13.5)
  line L316 (18.8107, 27.6837) -> (23, 24.1685)
  line L317 (23, 24.1685) -> (23, 13.5)
  line L318 (21.8255, 13.5) -> (23, 13.5)
  circle A35 centre (-25.5, 18.5) radius 0.475 construction
  circle A36 centre (-25.5, 18.5) radius 0.8
  circle A37 centre (-25.5, 18.5) radius 1.5
  circle A38 centre (25.5, 18.5) radius 0.8
  circle A39 centre (25.5, 18.5) radius 1.5
  circle A40 centre (25.5, 18.5) radius 0.475 construction
  line L319 (-11.6044, 45) -> (11.6044, 45)
  line L320 (26.8721, 25.6471) -> (13.9987, 27.4563)
  line L321 (13.9987, 27.4563) -> (12.6765, 18.0488)
  line L322 (12.6765, 18.0488) -> (25.55, 16.2395)
  line L323 (25.55, 16.2395) -> (26.8721, 25.6471)
  line L324 (-23.5658, 29.3614) -> (-18.675, 28.3218) construction
  line L325 (-20.1879, 33.2287) -> (-25.4441, 8.5) construction
  line L326 (-11.6068, 41.9956) -> (-9.0022, 44.1811)
  line L327 (-9.0022, 44.1811) -> (-6.8167, 41.5765)
  line L328 (-6.8167, 41.5765) -> (-9.4213, 39.391)
  line L329 (-9.4213, 39.391) -> (-11.6068, 41.9956)
  line L330 (-11.6068, 41.9956) -> (-6.8167, 41.5765) construction
  line L331 (-9.0022, 44.1811) -> (-9.4213, 39.391) construction
  line L332 (11.6068, 41.9956) -> (9.0022, 44.1811)
  line L333 (9.0022, 44.1811) -> (6.8167, 41.5765)
  line L334 (6.8167, 41.5765) -> (9.4213, 39.391)
  line L335 (9.4213, 39.391) -> (11.6068, 41.9956)
  circle A41 centre (-9.2117, 41.7861) radius 1.05
  circle A42 centre (9.2117, 41.7861) radius 1.05
  point P0 (-90, -90)
  point P1 (90, -90)
  point P2 (-21.625, 0)
  point P3 (-6.7221, 43.8751)
  point P4 (-5.3815, 45)
  point P5 (0, 49.5156)
  point P6 (-21.625, 0)
  point P7 (-90, -90)
  point P8 (90, -90)
  point P9 (-5.3815, 45)
  point P10 (5.3815, 45)
  point P11 (11.325, 41.9709)
  point P12 (7.0985, 41.6012)
  point P13 (23.3435, 30.4073)
  point P14 (-8.558, 47.5563)
  point P15 (0, 46.6253)
  point P16 (18.8107, 27.6837)
  point P17 (0, 54.7373)
  point P18 (0, 45.5994)
  point P19 (-3.7853, 57.9135)
  point P20 (3.7853, 57.9135)
  dimension "d352" = 15
  dimension "d359" = 2.1
  dimension "d360" = 2.1
  dimension "d361" = 2.1
  dimension "d362" = 2.1
  dimension "d405" = 1
  dimension "d410" = 1
  dimension "d411" = 6
  dimension "d412" = 20
  dimension "d413" = 5
  dimension "d414" = 1.5
  dimension "d422" = 12
  dimension "d426" = 5
  dimension "d427" = 4
  dimension "d428" = 5
  dimension "d430" = 5
  dimension "d432" = 50
  dimension "d434" = 4
  dimension "d435" = 4
  dimension "d436" = 130
  dimension "d437" = 18
  dimension "d438" = 4
  dimension "d439" = 1.5
  dimension "d451" = 4
  dimension "d466" = 5
  dimension "d467" = 45
  dimension "d468" = 4
  dimension "d469" = 5
  dimension "d470" = 3
  dimension "d471" = 6
  dimension "d491" = 1.25
  dimension "d492" = 1.6
  dimension "d497" = 3
  dimension "d499" = 3
  dimension "d503" = 1.25
  dimension "d504" = 1.6
  dimension "d505" = 3
  dimension "d506" = 3.5
  dimension "d507" = 9
  dimension "d509" = 1.6
  dimension "d510" = 3
  dimension "d515" = 1.5
  dimension "d516" = 1.5
  dimension "d517" = 2.25
  dimension "d518" = 2.25
  dimension "d520" = 5
  dimension "d521" = 5
  dimension "d532" = 0.95
  dimension "d533" = 1.6
  dimension "d534" = 3
  dimension "d538" = 2.5
  dimension "d539" = 5
  dimension "d546" = 78.5563
  dimension "d547" = 9.5
  dimension "d548" = 13
  dimension "d549" = 47.5563
  dimension "d552" = 2
  dimension "d556" = 0.2
  dimension "d557" = 0.2
  dimension "d560" = 2.1
  constraints: 178 end point, 49 horizontal alignment, 30 centre point, 23 point on line, 21 coincident, 20 parallel, 12 equal radius, 9 perpendicular, 8 collinear, 4 midpoint, 2 horizontal, 1 equal length, 1 tangent, 1 vertical, 43 other
  measures "d352" diameter of A12
  measures "d359" diameter of A13
  measures "d360" diameter of A14
  measures "d361" diameter of A15
  measures "d362" diameter of A16
  measures "d405" distance from line of L265 L110.start
  measures "d410" distance between parallel lines of L268 L265
  measures "d411" distance of L266.end L267.start
  measures "d412" angle of L267 L265
  measures "d413" distance between parallel lines of L270 L265
  measures "d414" distance between parallel lines of L271 L100
  measures "d422" angle of L161 L272
  measures "d426" distance between parallel lines of L272 L275
  measures "d428" distance between parallel lines of L280 L238
  measures "d432" angle of L158 L237
  measures "d434" distance of L158.start L282.end
  measures "d435" distance of L158.end L284.end
  measures "d436" angle of L286 L287
  measures "d437" distance of L159.start L286.end
  measures "d438" distance of L237.end L290.start
  measures "d439" distance between parallel lines of L160 L291
  measures "d451" distance between parallel lines of L283 L281
  measures "d466" distance between parallel lines of L159 L296
  measures "d467" angle of L297 L277
  measures "d468" distance of L295.end L296.end
  measures "d469" distance between parallel lines of L302 L231
  measures "d470" distance of L301.end L302.end
  measures "d471" distance of L278.start L303.end
  measures "d491" diameter of A18
  measures "d492" diameter of A19
  measures "d497" diameter of A20
  measures "d499" distance from line of L278 A18.centre
  measures "d503" diameter of A24
  measures "d504" diameter of A25
  measures "d505" diameter of A26
  measures "d506" distance from line of L277 A24.centre
  measures "d509" diameter of A30
  measures "d510" diameter of A31
  measures "d515" distance between parallel lines of L250 L309
  measures "d516" distance between parallel lines of L311 L243
  measures "d517" distance between parallel lines of L246 L310
  measures "d518" distance between parallel lines of L308 L258
  measures "d520" distance between parallel lines of L313 L287
  measures "d521" distance between parallel lines of L161 L314
  measures "d532" diameter of A35
  measures "d533" diameter of A36
  measures "d534" diameter of A37
  measures "d538" distance from line of L161 A35.centre
  measures "d539" distance from line of L315 A35.centre
  measures "d546" distance between parallel lines of L238 L265
  measures "d547" distance between parallel lines of L310 L308
  measures "d548" distance between parallel lines of L309 L311
  measures "d549" distance of the line from the sketch origin of L265
  measures "d552" distance from line of L324 L271.start
  measures "d556" distance between parallel lines of L98 L326
  measures "d557" distance between parallel lines of L329 L102
  measures "d560" diameter of A41
extrude "押し出し10" add sketch "スケッチ5" against normal blind 1 contours L272 A37 L311 L310 L314 L315 L296 L297 L309 L277 L300 L321 L322 L299 L318 L317 L323 A39 L274 L233 L235 L234 L284 L285 L238 L292 L291 L290 L283 L282 L231 L232 L230 | L272 A36 L311 A37 | L272 L311 A36 | A37 L260 L314 L310 L311 | L311 A36 L272 A37 L248 L260 | L272 L273 L319 L294 L274 L320 L316 L276 L293 L270 L271 L275 L313 L308 | L272 A36 L311 | L272 L248 A37 | L308 L313 L314 L258 L272 | L272 L258 L314 L260 A37 L248 | A37 L260 L248 | L314 L260 L275 L295 L310 | L310 L295 L315 L314 | L267 L268 L269 | L273 L265 L267 L269 L294 L319 | L313 L275 L308 | L308 L275 L258 L314 L313 | L310 L297 L296 L295 | L295 L277 L309 L297 L310 | L314 L258 L275 L260 | L308 L309 L277 L275 L260 L259 L258 | L275 L271 L270 L293 L276 L320 L321 L277 L309 L308 | L290 L291 L292 L238 | L297 L309 L310 | L275 L258 L259 L260 | L265 L269 L267 | L277 L297 L309 | L274 L261 L317 L316 L320 | L277 L321 L300 | L274 L262 A39 L263 L317 L261 | L320 L276 L316 | L316 L317 L261 L276 L320 | L321 L320 L276 L261 L264 L263 L277 | L277 L298 L322 L300 L321 | L300 L322 L321 | L317 L263 L276 L261 | L274 A39 L262 | A39 L323 A38 L274 | L276 L263 L317 L322 L298 | L322 L298 L299 L300 | L276 L263 L264 L261 | L263 A39 L323 L322 L317 | A39 L274 A38 L323 L263 L262 | L262 L263 A39 | A38 L323 L274 | L322 L317 L318 L298 | L274 L323 A38 | A12 | A13 | A14 | A15 | A16 | L301 L302 L303 L278 | L278 L279 L280 L281 | L306 L305 L304 L278 | A19 | A20 | A22 | A23 | A25 | A26 | A28 | A29 | A30 | A33 | L326 L327 L328 L329 | L335 L334 L333 L332 | A41 | A42 picked at (-25.7501, 17.2631) picked at (-25.8266, 18.0143) picked at (-25.0976, 18.4435) picked at (25.7501, 17.2631) picked at (25.8266, 18.0143) picked at (25.0946, 18.4887)
extrude "押し出し11" cut sketch "スケッチ5" against normal blind 1.5 contours L310 L297 L296 L295 | L295 L277 L309 L297 L310 | L277 L297 L309 | L277 L321 L300 | L277 L298 L322 L300 L321 | L322 L298 L299 L300 | L301 L302 L303 L278 | L306 L305 L304 L278
chamfer "面取り8" distance 2 angle 45 2 edges at (-21.8255, 13.5, -0.5) (21.8255, 13.5, -0.5)